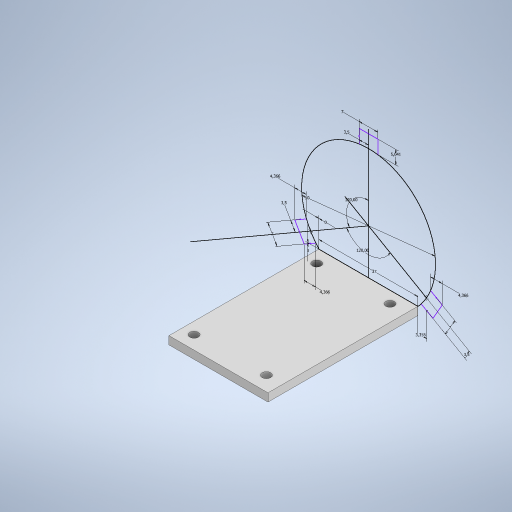
# Autodesk Inventor part: Electronic casing
Saved by Autodesk Inventor 2024 (Build 280153000, 153)
## iProperties
Created: 2024-03-27
Part Number: Electronic casing
Material: Generic
Document SubType Name: Modeling
Designer: auror
Density: 1 g/cm^3
Appearance: Default
Author: auror
Autodesk Inventor part; units mm, degrees
ref_plane "YZ Plane" through (0, 0, 0) normal (1, 0, 0) x (0, 1, 0)
ref_plane "XZ Plane" through (0, 0, 0) normal (0, 1, 0) x (-1, 0, 0)
ref_plane "XY Plane" through (0, 0, 0) normal (0, 0, 1) x (1, 0, 0)
sketch "Sketch2" plane through (0, 0, 0) normal (0, 1, 0) x (-1, 0, 0)
  line L0 (18.5, 28) -> (-18.5, 28)
  line L1 (-18.5, 28) -> (-18.5, -28)
  line L2 (-18.5, -28) -> (18.5, -28)
  line L3 (18.5, -28) -> (18.5, 28)
  point P0 (0, 0)
  point P1 (-18.5, 0)
  point P2 (18.5, 0)
  dimension "d0" = 37
  dimension "d1" = 56
  dimension "d2" = 28
  dimension "d3" = 18.5
  constraints: 8 end point, 2 midpoint, 2 parallel, 1 horizontal, 1 perpendicular
  measures "d0" distance of point (-18.5, 0) point (18.5, 0)
  measures "d1" distance between parallel lines of L2 L0
  measures "d2" distance from line of point (0, 0) L0
  measures "d3" distance from line of L3 point (0, 0)
extrude "Extrusion1" add sketch "Sketch2" along normal blind 3
sketch "Sketch3" plane through (0, 3, 0) normal (0, 1, 0) x (1, 0, 0)
  circle A0 centre (12.5, -22.6) radius 1.6
  circle A1 centre (-14.1006, -23.0348) radius 1.6
  circle A2 centre (-14.2118, 22.9033) radius 1.6
  circle A3 centre (12.5, 23.5707) radius 1.6
  point P0 (0, 0)
  dimension "d6" = 22.6
  dimension "d7" = 12.5
  dimension "d8" = 3.2
  dimension "d9" = 3.2
  dimension "d10" = 3.2
  dimension "d11" = 3.2
  constraints: 4 centre point, 4 coincident
  measures "d6" vertical distance of point (0, 0) point (12.5, -22.6)
  measures "d7" horizontal distance of point (0, 0) point (12.5, -22.6)
  measures "d8" diameter of A0
  measures "d9" diameter of A1
  measures "d10" diameter of A2
  measures "d11" diameter of A3
hole "Hole1" at (12.5, 3, 22.6) at (-14.1006, 3, 23.0348) at (-14.2118, 3, -22.9033) at (12.5, 3, -23.5707) direction (0, -1, 0) diameter 3.2 end through all
sketch "Sketch4" plane through (18.5, 0, -28) normal (0, 0, -1) x (-1, 0, 0)
  circle A0 centre (18.5, 19.8152) radius 25
  line L0 (0, 3) -> (37, 3)
  line L1 (0, 3) -> (37, 3) projected
  line L2 (18.5, 44.8152) -> (18.5, 3)
  line L3 (18.5, 19.8152) -> (-3.1506, 7.3152)
  line L4 (18.5, 19.8152) -> (18.5, 44.8152)
  line L5 (18.5, 19.8152) -> (40.1506, 7.3152)
  line L6 (15, 49.6103) -> (15, 44.569)
  line L7 (22, 49.6103) -> (22, 44.569)
  line L8 (15, 49.6103) -> (22, 49.6103)
  line L9 (-9.0441, 7.9828) -> (-4.678, 10.446)
  line L10 (-5.5382, 1.9245) -> (-1.1716, 4.387)
  line L11 (-9.0441, 7.9828) -> (-5.5382, 1.9245)
  line L12 (41.6874, 10.4694) -> (46.0533, 7.9487)
  line L13 (38.1874, 4.4072) -> (42.5533, 1.8865)
  line L14 (42.5533, 1.8865) -> (46.0533, 7.9487)
  line L15 (18.5, 19.8152) -> (-3.1506, 7.3152)
  line L16 (27.2924, 24.8915) -> (-3.1506, 7.3152)
  line L17 (18.5, 19.8152) -> (18.5, 44.8152)
  line L18 (18.5, 51.0394) -> (18.5, 44.8152)
  line L19 (18.5, 19.8152) -> (40.1506, 7.3152)
  line L20 (85.0332, -18.5978) -> (40.1506, 7.3152)
  point P0 (18.5, 0)
  point P1 (-3.3549, 3.1558)
  point P2 (40.3704, 3.1469)
  point P3 (-6.861, 9.2144)
  point P4 (22, 47.0896)
  point P5 (43.8704, 9.209)
  dimension "d19" = 50
  dimension "d20" = 37
  dimension "d21" = 120
  dimension "d22" = 120
  dimension "d32" = 7
  dimension "d33" = 7
  dimension "d34" = 7
  dimension "d35" = 0
  dimension "d36" = 3.3549
  dimension "d37" = 3.5
  dimension "d38" = 3.5
  dimension "d39" = 3.5
  dimension "d40" = 5.0414
  dimension "d41" = 4.3661
  dimension "d42" = 4.3659
  dimension "d43" = 4.3659
  dimension "d44" = 0
  constraints: 40 end point, 6 collinear, 6 midpoint, 3 point on line, 1 coincident, 1 perpendicular, 1 vertical, 13 other
  measures "d20" distance of L0.start L0.end
  measures "d32" distance of point (-3.355, 3.156) point (-6.861, 9.214)
  measures "d33" distance from line of point (22, 47.09) L6
  measures "d34" distance of point (43.87, 9.209) point (40.37, 3.147)
  measures "d35" distance between parallel lines of L1 L0
  measures "d36" horizontal distance of point (-3.355, 3.156) L0.start
  measures "d37" distance from line of L16 point (-3.355, 3.156)
  measures "d38" distance from line of point (22, 47.09) L18
  measures "d39" distance from line of L20 point (43.87, 9.209)
  measures "d40" distance of L6.start L6.end
  measures "d41" horizontal distance of L9.start L9.end
  measures "d42" horizontal distance of L12.start L12.end
  measures "d43" horizontal distance of L13.start L13.end
  measures "d44" distance of L1.end L0.end
body "Solid1"
